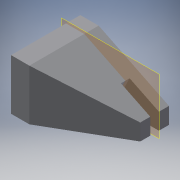
# Autodesk Inventor part: Importing AutoCAD Geometry
Saved by Autodesk Inventor 2016 (Build 200138000, 138)
## iProperties
Created: 2013-12-03
Part Number: Importing AutoCAD Geometry
Material: Generic
Document SubType Name: Modeling
Designer: John
Density: 1 g/cm^3
Appearance: Default
Author: John
Autodesk Inventor part; units mm, degrees
ref_plane "YZ Plane" through (0, 0, 0) normal (1, 0, 0) x (0, 1, 0)
ref_plane "XZ Plane" through (0, 0, 0) normal (0, 1, 0) x (-1, 0, 0)
ref_plane "XY Plane" through (0, 0, 0) normal (0, 0, 1) x (1, 0, 0)
sketch "Sketch1" plane through (0, 0, 0) normal (0, 0, 1) x (1, 0, 0)
  line L0 (0, 0) -> (32.4623, 0)
  line L1 (32.4623, 0) -> (32.4623, 18.6079)
  line L2 (32.4623, 18.6079) -> (0, 18.6079)
  line L3 (0, 18.6079) -> (0, 0)
  constraints: 8 end point, 2 parallel, 1 horizontal, 1 perpendicular
extrude "Extrusion1" add sketch "Sketch1" along normal blind 25.4
sketch "Sketch2" plane through (0, 0, 25.4) normal (0, 0, 1) x (1, 0, 0)
  line L0 (32.4623, 0) -> (32.4623, 18.6079) projected
  line L1 (32.4623, 18.6079) -> (0, 18.6079) projected
  line L2 (6.7125, 18.6079) -> (32.4623, 6.0135)
  constraints: 2 end point, 2 point on line
extrude "Extrusion2" cut sketch "Sketch2" against normal through all
sketch "Sketch4" plane through (0, 18.6079, 25.4) normal (0, 1, 0) x (1, 0, 0)
  line L0 (0, 25.4) -> (0, 0) projected
  line L1 (6.7125, 25.4) -> (32.4623, 25.4) projected
  line L2 (6.7125, 0) -> (6.7125, 25.4) projected
  line L3 (32.4623, 0) -> (6.7125, 0) projected
  line L4 (32.4623, 25.4) -> (32.4623, 0) projected
  line L5 (6.7125, 0) -> (32.4623, 14.8667)
  dimension "d6" = 30
  constraints: 2 end point, 1 point on line
  measures "d6" angle of L3 L5
extrude "Extrusion4" cut sketch "Sketch4" against normal through all contours L5 L4 L3
ref_plane "Work Plane1" through (32.4623, 6.0135, 5.2667) normal (0, 0, 1) x (1, 0, 0)
sketch "Sketch5" plane through (32.4623, 6.0135, 5.2667) normal (0, 0, 1) x (1, 0, 0)
  line L0 (-32.4623, -6.0135) -> (-32.4623, 12.5943) projected
  line L1 (-32.4623, 12.5943) -> (-25.7498, 12.5943) projected
  line L2 (-25.7498, 12.5943) -> (0, 0) projected
  line L3 (0, 0) -> (0, -6.0135) projected
  line L4 (0, -6.0135) -> (-32.4623, -6.0135) projected
  line L5 (-16.2312, -6.0135) -> (-10.7244, 5.2453)
  constraints: 2 end point, 1 midpoint, 1 perpendicular, 1 point on line
extrude "Extrusion5" cut sketch "Sketch5" along normal mid plane 3.175 contours L5 L2 L3 L4
body "Solid1"
